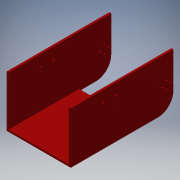
# Autodesk Inventor part: Base Bucket
Saved by Autodesk Inventor 2016 (Build 200138000, 138)
## iProperties
Created: 2015-12-16
Part Number: Base Bucket
Material: Generic
Document SubType Name: Modeling
Designer: TimB
Density: 1 g/cm^3
Appearance: Red
Author: TimB
Autodesk Inventor part; units mm, degrees
ref_plane "YZ Plane" through (0, 0, 0) normal (1, 0, 0) x (0, 1, 0)
ref_plane "XZ Plane" through (0, 0, 0) normal (0, 1, 0) x (-1, 0, 0)
ref_plane "XY Plane" through (0, 0, 0) normal (0, 0, 1) x (1, 0, 0)
sketch "Sketch1" plane through (0, 0, 0) normal (0, 1, 0) x (-1, 0, 0)
  line L0 (-63.5, -101.6) -> (63.5, -101.6)
  line L1 (63.5, -101.6) -> (63.5, 101.6)
  line L2 (63.5, 101.6) -> (-63.5, 101.6)
  line L3 (-63.5, 101.6) -> (-63.5, -101.6)
  line L4 (-63.5, -101.6) -> (63.5, 101.6) construction
  line L5 (63.5, -101.6) -> (-63.5, 101.6) construction
  point P0 (0, 0)
  dimension "d0" = 127
  dimension "d1" = 203.2
  constraints: 12 end point, 2 midpoint, 2 parallel, 1 horizontal, 1 perpendicular
  measures "d0" distance of L2.end L1.end
  measures "d1" distance of L1.end L0.end
extrude "Extrusion1" add sketch "Sketch1" along normal blind 101.6
sketch "Sketch3" plane through (0, 101.6, 0) normal (0, 1, 0) x (1, 0, 0)
  line L0 (63.5, 101.6) -> (-63.5, 101.6) projected
  line L1 (59.69, -101.6) -> (-59.69, -101.6)
  line L2 (-59.69, -101.6) -> (-59.69, 101.6)
  line L3 (-59.69, 101.6) -> (59.69, 101.6)
  line L4 (59.69, 101.6) -> (59.69, -101.6)
  line L5 (59.69, -101.6) -> (-59.69, 101.6) construction
  line L6 (-59.69, -101.6) -> (59.69, 101.6) construction
  point P0 (0, 0)
  dimension "d4" = 119.38
  constraints: 12 end point, 2 midpoint, 2 parallel, 1 horizontal, 1 perpendicular, 1 point on line
  measures "d4" distance of L2.end L3.end
extrude "Extrusion2" cut sketch "Sketch3" against normal blind 97.79
sketch "Sketch4" plane through (0, 3.81, 0) normal (0, 1, 0) x (1, 0, 0)
  line L0 (59.69, 101.6) -> (59.69, -101.6) projected
  line L1 (-59.69, 101.6) -> (59.69, 101.6) projected
  line L2 (59.69, 101.6) -> (-59.69, 101.6)
  line L3 (-59.69, 101.6) -> (-59.69, 38.1)
  line L4 (-59.69, 38.1) -> (59.69, 38.1)
  line L5 (59.69, 38.1) -> (59.69, 101.6)
  point P0 (0, 0)
  dimension "d7" = 63.5
  constraints: 8 end point, 3 equal length, 1 perpendicular
  measures "d7" distance of L3.end L1.start
extrude "Extrusion3" cut sketch "Sketch4" against normal blind 3.81
fillet "Fillet1" radius 30.48 2 edges at (61.595, 0, -101.6) (-61.595, 0, -101.6)
sketch "Sketch7" plane through (63.5, 0, 101.6) normal (1, 0, 0) x (0, 0, -1)
  circle A0 centre (189.7, 55.45) radius 1.85 projected
  circle A1 centre (197.7, 47.45) radius 1.85 projected
  circle A2 centre (181.7, 47.45) radius 1.85 projected
  circle A3 centre (189.7, 39.45) radius 1.85 projected
  point P0 (101.6, 0)
hole "Hole2" at (63.5, 55.45, -88.1) at (63.5, 47.45, -96.1) at (63.5, 47.45, -80.1) at (63.5, 39.45, -88.1) direction (-1, 0, 0) diameter 3.7 end through all
sketch "Sketch8" plane through (63.5, 0, 101.6) normal (1, 0, 0) x (0, 0, -1)
  circle A0 centre (63.5, 80.01) radius 1.85 projected
  circle A1 centre (88.9, 80.01) radius 1.85 projected
  point P0 (101.6, 0)
hole "Hole3" at (63.5, 80.01, 38.1) at (63.5, 80.01, 12.7) direction (-1, 0, 0) diameter 3.7 end through all
body "Solid1"
